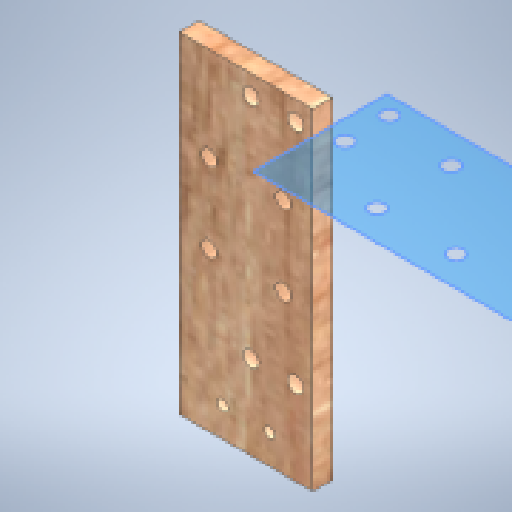
# Autodesk Inventor part: фанера_каретка
Saved by Autodesk Inventor 2023.1 (Build 271208000, 208)
## iProperties
Created: 2026-01-04
Part Number: фанера_каретка
Material: Древесина (береза)
Document SubType Name: Modeling
Designer: DELL
Density: 0.55 g/cm^3
Appearance: Береза — натуральный — полированный
Author: DELL
Autodesk Inventor part; units mm, degrees
ref_plane "YZ Plane" through (0, 0, 0) normal (1, 0, 0) x (0, 1, 0)
ref_plane "XZ Plane" through (0, 0, 0) normal (0, 1, 0) x (-1, 0, 0)
ref_plane "XY Plane" through (0, 0, 0) normal (0, 0, 1) x (1, 0, 0)
sketch "Эскиз1" plane through (0, 0, 0) normal (0, 0, 1) x (1, 0, 0)
  circle A0 centre (-7.5, -6.95) radius 1.5 construction
  circle A1 centre (7.5, -6.95) radius 1.5 construction
  circle A2 centre (7.5, -22.95) radius 1.5 construction
  circle A3 centre (-7.5, -22.95) radius 1.5 construction
  circle A4 centre (-7.5, -6.95) radius 1.6
  circle A5 centre (7.5, -6.95) radius 1.6
  circle A6 centre (7.5, -22.95) radius 1.6
  circle A7 centre (-7.5, -22.95) radius 1.6
  line L0 (9, 4.1) -> (-9, 4.1) construction
  line L1 (9, -34) -> (-9, -34) construction
  line L2 (-13.5, 12.05) -> (13.5, 12.05)
  line L3 (13.5, 12.05) -> (13.5, -41.95)
  line L4 (13.5, -41.95) -> (-13.5, -41.95)
  line L5 (-13.5, -41.95) -> (-13.5, 12.05)
  line L6 (-7.5, -6.95) -> (-7.5, 12.05) construction
  line L7 (-7.5, -22.95) -> (-7.5, -41.95) construction
  point P0 (0, 0)
  dimension "d0" = 3.2
  dimension "d1" = 3.2
  dimension "d2" = 3.2
  dimension "d3" = 3.2
  dimension "d4" = 6
  dimension "d5" = 6
  dimension "d8" = 54
  constraints: 12 end point, 4 centre point, 4 coincident, 3 point on line, 2 parallel, 2 perpendicular, 1 collinear, 1 horizontal
  measures "d0" diameter of A4
  measures "d1" diameter of A5
  measures "d2" diameter of A6
  measures "d3" diameter of A7
  measures "d4" distance from line of L3 A5.centre
  measures "d5" distance from line of L5 A0.centre
  measures "d8" distance between parallel lines of L4 L2
extrude "Выдавливание1" add sketch "Эскиз1" along normal blind 4
sketch "Эскиз3" plane through (0, 0, 4) normal (0, 0, 1) x (1, 0, 0)
  circle A0 centre (1, -37.95) radius 2.1 construction
  circle A1 centre (10, -37.95) radius 2.1 construction
  circle A2 centre (1, 8.05) radius 2.1 construction
  circle A3 centre (10, 8.05) radius 2.1 construction
  circle A4 centre (1, -37.95) radius 1.6
  circle A5 centre (10, -37.95) radius 1.6
  circle A6 centre (1, 8.05) radius 1.6
  circle A7 centre (10, 8.05) radius 1.6
  point P0 (0, 0)
  dimension "d9" = 3.2
  dimension "d10" = 3.2
  dimension "d11" = 3.2
  dimension "d12" = 3.2
  constraints: 4 centre point, 4 coincident
  measures "d9" diameter of A4
  measures "d10" diameter of A5
  measures "d11" diameter of A7
  measures "d12" diameter of A6
extrude "Выдавливание2" cut sketch "Эскиз3" against normal blind 10
sketch "Эскиз4" plane through (-13.5, -41.95, 0) normal (0, -1, 0) x (1, 0, 0)
  line L0 (0, 4) -> (27, 4) projected
  line L1 (0, 0) -> (0, 4) projected
  line L2 (0, 0) -> (27, 0) projected
  line L3 (27, 0) -> (27, 4) projected
  point P0 (13.5, 0)
extrude "Выдавливание3" add sketch "Эскиз4" along normal blind 13
sketch "Эскиз5" plane through (0, 0, 4) normal (0, 0, 1) x (1, 0, 0)
  circle A0 centre (-4.75, -48.95) radius 1.1
  circle A1 centre (4.75, -48.95) radius 1.1
  line L0 (13.5, -54.95) -> (-13.5, -54.95) projected
  line L1 (-4.75, -48.95) -> (4.75, -48.95) construction
  line L2 (-13.5, -54.95) -> (13.5, -54.95) projected
  line L3 (0, -54.95) -> (0, -44.9409) construction
  point P0 (0, 0)
  point P1 (0, -48.95)
  dimension "d17" = 2.2
  dimension "d18" = 2.2
  dimension "d19" = 6
  dimension "d20" = 6
  dimension "d21" = 9.5
  constraints: 4 end point, 2 centre point, 2 midpoint, 1 point on line, 1 vertical
  measures "d17" diameter of A0
  measures "d18" diameter of A1
  measures "d19" distance from line of L0 L1.start
  measures "d20" distance from line of L0 L1.end
  measures "d21" distance of L1.start L1.end
extrude "Выдавливание4" cut sketch "Эскиз5" against normal blind 13
